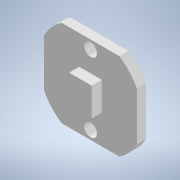
# Autodesk Inventor part: AS5600
Saved by Autodesk Inventor 2022 (Build 260153070, 153G)
## iProperties
Created: 2021-10-29
Part Number: AS5600
Material: Generic
Document SubType Name: Modeling
Designer: a laptop
Density: 1 g/cm^3
Appearance: Default
Author: a laptop
Autodesk Inventor part; units mm, degrees
ref_plane "YZ Plane" through (0, 0, 0) normal (1, 0, 0) x (0, 1, 0)
ref_plane "XZ Plane" through (0, 0, 0) normal (0, 1, 0) x (-1, 0, 0)
ref_plane "XY Plane" through (0, 0, 0) normal (0, 0, 1) x (1, 0, 0)
sketch "Sketch1" plane through (0, 0, 0) normal (0, 0, 1) x (1, 0, 0)
  line L0 (8, 7.5) -> (4.9749, 7.5) construction
  line L1 (-8, 7.5) -> (-8, 4.1231) construction
  line L2 (-8, -7.5) -> (-4.9749, -7.5) construction
  line L3 (8, -7.5) -> (8, -4.1231) construction
  arc A0 (8, 4.1231) -> (4.9749, 7.5) centre (0, 0) ccw
  arc A1 (8, -4.1231) -> (8, 4.1231) centre (0, 0) ccw construction
  arc A2 (-4.9749, 7.5) -> (-8, 4.1231) centre (0, 0) ccw
  arc A3 (-4.9749, -7.5) -> (4.9749, -7.5) centre (0, 0) ccw construction
  arc A4 (4.9749, -7.5) -> (8, -4.1231) centre (0, 0) ccw
  line L4 (4.9749, -7.5) -> (8, -7.5) construction
  line L5 (-4.9749, -7.5) -> (4.9749, -7.5)
  line L6 (-8, -4.1231) -> (-8, -7.5) construction
  line L7 (8, 4.1231) -> (8, 7.5) construction
  line L8 (8, -4.1231) -> (8, 4.1231)
  line L9 (-8, 4.1231) -> (-8, -4.1231)
  line L10 (-4.9749, 7.5) -> (-8, 7.5) construction
  arc A5 (4.9749, 7.5) -> (-4.9749, 7.5) centre (0, 0) ccw construction
  arc A6 (-8, 4.1231) -> (-8, -4.1231) centre (0, 0) ccw construction
  arc A7 (-8, -4.1231) -> (-4.9749, -7.5) centre (0, 0) ccw
  line L11 (4.9749, 7.5) -> (-4.9749, 7.5)
  circle A8 centre (0, -6) radius 1.1
  circle A9 centre (0, 6) radius 1.1
  dimension "d3" = 15
  dimension "d4" = 16
  dimension "d6" = 7.5
  dimension "d7" = 8
  dimension "d8" = 18
  dimension "d9" = 6
  dimension "d10" = 2.2
  dimension "d11" = 2.2
  dimension "d12" = 6
  constraints: 24 end point, 18 parallel, 17 point on circle, 10 centre point, 9 perpendicular, 3 horizontal, 2 vertical alignment, 1 coincident
  measures "d3" distance of L3.start L0.start
  measures "d4" distance of L2.start L3.start
  measures "d6" distance from line of L0 point (0, 0)
  measures "d7" distance from line of L3 point (0, 0)
  measures "d8" diameter of A0
  measures "d9" distance of point (0, 0) A8.centre
  measures "d10" diameter of A8
  measures "d11" diameter of A9
  measures "d12" distance of point (0, 0) A9.centre
extrude "Extrusion1" add sketch "Sketch1" along normal blind 1.57
sketch "Sketch2" plane through (0, 0, 1.57) normal (0, 0, 1) x (1, 0, 0)
  line L0 (1.95, 2.45) -> (-1.95, 2.45)
  line L1 (-1.95, 2.45) -> (-1.95, -2.45)
  line L2 (-1.95, -2.45) -> (1.95, -2.45)
  line L3 (1.95, -2.45) -> (1.95, 2.45)
  point P0 (0, 0)
  dimension "d15" = 4.9
  dimension "d16" = 3.9
  dimension "d17" = 1.95
  dimension "d18" = 2.45
  constraints: 8 end point, 2 parallel, 1 horizontal, 1 perpendicular
  measures "d15" distance of L2.end L0.start
  measures "d16" distance of L1.end L2.end
  measures "d17" distance from line of L3 point (0, 0)
  measures "d18" distance from line of point (0, 0) L0
extrude "Extrusion2" add sketch "Sketch2" along normal blind 1.75
body "Solid1"
